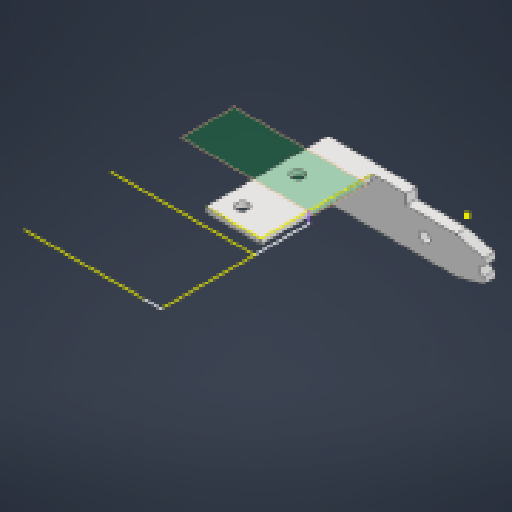
# Autodesk Inventor part: Bridge
Saved by Autodesk Inventor 2027.1 (Build 311270010, 270A)
## iProperties
Created: 2026-10-05
Part Number: Bridge
Material: Generic
Document SubType Name: Modeling
Designer: prkr
Density: 1 g/cm^3
Appearance: Default
Author: prkr
Autodesk Inventor part; units mm, degrees
ref_plane "YZ Plane" through (0, 0, 0) normal (1, 0, 0) x (0, 1, 0)
ref_plane "XZ Plane" through (0, 0, 0) normal (0, 1, 0) x (-1, 0, 0)
ref_plane "XY Plane" through (0, 0, 0) normal (0, 0, 1) x (1, 0, 0)
sketch "Sketch1" plane through (0, 0, 0) normal (0, 0, 1) x (1, 0, 0)
  circle A0 centre (7.5, 0) radius 1.15 projected
  circle A1 centre (7.5, 0) radius 0.95 projected
  circle A2 centre (-8.5, 0) radius 1.5 construction
  circle A3 centre (7.5, 0) radius 1.3
  circle A4 centre (-8.5, 0) radius 1.4
  line L0 (7.5, -1.3) -> (7.5, -3)
  line L1 (7.5, -3) -> (0.0359, -5)
  line L2 (0.0359, -5) -> (-13.5, -5)
  line L3 (7.5, -1.3) -> (7.5, 0)
  line L4 (-13.5, -5) -> (-13.5, 0)
  line L5 (-13.5, 0) -> (7.5, 0)
  line L6 (-22.6, 7.7551) -> (-58.6, 7.7551) projected
  line L7 (-22.6, 7.7551) -> (-13.5, 7.7551)
  line L8 (-13.5, 7.7551) -> (-13.5, 0)
  point P0 (0, 0)
  point P1 (6.2, 0)
  point P2 (-7.1, 0)
  point P3 (-9.9, 0)
  dimension "d1" = 0.15
  dimension "d2" = 5
  dimension "d3" = 15
  dimension "d4" = 3
  dimension "d5" = 5
  dimension "d8" = 2.8
  constraints: 16 end point, 3 perpendicular, 3 vertical, 2 coincident, 1 centre point, 1 collinear, 3 other
  measures "d2" distance from line of L2 A4.centre
  measures "d3" angle of L2 L1
  measures "d4" distance of A0.centre L0.end
  measures "d5" distance of L4.end A2.centre
  measures "d8" diameter of A4
extrude "Extrusion1" add sketch "Sketch1" along normal blind 3 contours A3 L0 L1 L2 L4 L5 A4
mirror "Mirror1" about plane through (6.2, 0, 0) normal (0, 1, 0) of "Extrusion1"
ref_plane "Work Plane1" through (-19.6, 7.75, 6.7) normal (0, -1, 0) x (-1, 0, 0)
sketch "Sketch2" plane through (-19.6, 7.75, 6.7) normal (0, -1, 0) x (-1, 0, 0)
  circle A0 centre (13, -6.5) radius 1.25 construction
  circle A1 centre (13, -21.5) radius 1.5 construction
  circle A2 centre (13, -6.5) radius 1.7
  circle A3 centre (13, -21.5) radius 1.7
  line L0 (18, 6.7) -> (18, -26.5)
  line L1 (18, -26.5) -> (8, -26.5)
  line L2 (3, 6.7) -> (39, 6.7) projected
  line L3 (-6.1, 6.7) -> (-6.1, 3.7) projected
  line L4 (-6.1, 3.7) -> (-19.6359, 3.7) projected
  line L5 (-6.1, 3.7) -> (8, 3.7)
  line L6 (8, 3.7) -> (8, -26.5)
  line L7 (8, 3.7) -> (18, 3.7)
  line L8 (3, 6.7) -> (-6.1, 6.7) projected
  line L9 (8.5, -12.5) -> (8.5, -3) projected
  line L10 (3, 0) -> (3, -2.5) projected
  point P0 (-19.6, 6.7)
  dimension "d9" = 3.4
  dimension "d10" = 5
  dimension "d11" = 5
  dimension "d12" = 5
  constraints: 10 end point, 2 centre point, 2 coincident, 2 perpendicular, 1 equal radius, 1 horizontal, 1 parallel, 1 point on line, 1 vertical
  measures "d9" diameter of A2
  measures "d10" distance from line of L0 A0.centre
  measures "d11" distance from line of L1 A1.centre
  measures "d12" distance from line of A1.centre L6
extrude "Extrusion2" add sketch "Sketch2" along normal up to surface (12.75 mm away) contours L0 L7 L5 L3 L8 L2
sketch "Sketch3" plane through (-19.6, 7.75, 6.7) normal (0, -1, 0) x (-1, 0, 0)
  line L0 (18, 3.7) -> (-19.6359, 3.7) projected
  line L1 (18, 3.7) -> (18, -26.5)
  line L2 (18, -26.5) -> (3, -26.5)
  line L3 (3, -26.5) -> (3, 3.7)
  line L4 (3, 3.7) -> (18, 3.7)
  line L5 (3, 0) -> (3, -2.5) projected
  line L6 (18, -26.5) -> (8, -26.5) projected
  circle A0 centre (13, -6.5) radius 1.7 projected
  circle A1 centre (13, -21.5) radius 1.7 projected
  point P0 (-19.6, 6.7)
  point P1 (3, 3.7)
  constraints: 8 end point, 2 parallel, 1 perpendicular, 1 point on line, 1 vertical
extrude "Extrusion3" add sketch "Sketch3" along normal blind 1.5
sketch "Sketch4" plane through (-19.6, 7.75, 6.7) normal (0, -1, 0) x (-1, 0, 0)
  line L0 (3, -26.5) -> (18, -26.5) projected
  line L1 (37.1716, -56.5) -> (4.8284, -56.5) projected
  line L2 (0, -56) -> (0, -50.5) projected
  line L3 (4.8284, -56.5) -> (0, -56.5)
  line L4 (0, -56.5) -> (0, -56)
  line L5 (3, -31.2051) -> (39, -31.2051) projected
  line L6 (0, -37.5) -> (0, -31.5) projected
  line L7 (0, -50.5) -> (0, -37.5) projected
  line L8 (3, -31.2051) -> (0.0051, -31.2051) projected
  line L9 (0.0051, -31.2051) -> (0, -31.5)
  line L10 (0.0051, -31.2051) -> (0.0051, -16.6049)
  line L11 (0.0051, -16.6049) -> (3, -13)
  line L12 (3, 3.7) -> (3, -26.5) projected
  line L13 (3, -13) -> (0.3229, -13) projected
  line L14 (-0.1, -16.5) -> (-0.9, -16.5) projected
  line L15 (-0.1, -16.5) -> (0.0026, -16.5) construction
  point P0 (-19.6, 6.7)
  constraints: 12 end point, 2 horizontal, 1 perpendicular, 1 vertical
body "Solid1"
